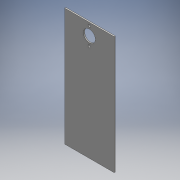
# Autodesk Inventor part: sholder_fin
Saved by Autodesk Inventor 2016 (Build 200138000, 138)
## iProperties
Created: 2016-11-19
Part Number: sholder_fin
Material: 一般
Document SubType Name: Modeling
Designer: 宏太
Density: 1 g/cm^3
Appearance: 既定
Author: 宏太
Autodesk Inventor part; units mm, degrees
ref_plane "YZ Plane" through (0, 0, 0) normal (1, 0, 0) x (0, 1, 0)
ref_plane "XZ Plane" through (0, 0, 0) normal (0, 1, 0) x (-1, 0, 0)
ref_plane "XY Plane" through (0, 0, 0) normal (0, 0, 1) x (1, 0, 0)
sketch "スケッチ1" plane through (0, 0, 0) normal (0, 1, 0) x (-1, 0, 0)
  line L0 (0, 0) -> (84, 0)
  line L1 (84, 0) -> (84, -200)
  line L2 (84, -200) -> (0, -200)
  line L3 (0, -200) -> (0, 0)
  dimension "d0" = 84
  dimension "d1" = 200
  constraints: 8 end point, 2 parallel, 1 horizontal, 1 perpendicular
  measures "d0" distance of L1.end L2.end
  measures "d1" distance of L0.end L1.end
extrude "押し出し1" add sketch "スケッチ1" along normal blind 2
sketch "スケッチ2" plane through (0, 2, 0) normal (0, 1, 0) x (1, 0, 0)
  circle A0 centre (-42, 5) radius 2.1
  line L0 (0, 0) -> (0, 200) projected
  line L1 (-84, 0) -> (0, 0) projected
  circle A1 centre (-42, 35) radius 2.1
  circle A2 centre (-42, 20) radius 10.1
  dimension "d4" = 4.2
  dimension "d5" = 42
  dimension "d6" = 5
  dimension "d7" = 4.2
  dimension "d8" = 30
  dimension "d11" = 20.2
  dimension "d12" = 15
  constraints: 3 centre point
  measures "d4" diameter of A0
  measures "d5" distance from line of L0 A0.centre
  measures "d6" distance from line of L1 A0.centre
  measures "d7" diameter of A1
  measures "d8" distance of A1.centre A0.centre
  measures "d11" diameter of A2
  measures "d12" distance of A1.centre A2.centre
extrude "押し出し3" cut sketch "スケッチ2" against normal blind 2
